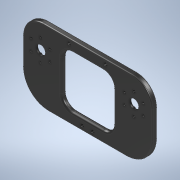
# Autodesk Inventor part: Fechamento_Corpo
Saved by Autodesk Inventor 2020 (Build 240168000, 168)
## iProperties
Created: 2021-05-17
Part Number: Fechamento_Corpo
Material: Plástico PC/ABS
Document SubType Name: Modeling
Designer: JCarlos
Density: 0.357273 g/cm^3
Appearance: Brilhosa - Preta
Author: JCarlos
Autodesk Inventor part; units mm, degrees
ref_plane "YZ Plane" through (0, 0, 0) normal (1, 0, 0) x (0, 1, 0)
ref_plane "XZ Plane" through (0, 0, 0) normal (0, 1, 0) x (-1, 0, 0)
ref_plane "XY Plane" through (0, 0, 0) normal (0, 0, 1) x (1, 0, 0)
sketch "Esboço1" plane through (0, 0, 0) normal (0, 0, 1) x (1, 0, 0)
  line L0 (42.5, 33) -> (-42.5, 33)
  line L1 (-62.5, 13) -> (-62.5, -13)
  line L2 (-37.5, -38) -> (37.5, -38)
  line L3 (62.5, -13) -> (62.5, 13)
  line L4 (-15, 22.5) -> (15, 22.5)
  arc A0 (-15, 22.5) -> (-25, 12.5) centre (-15, 12.5) ccw
  line L5 (-25, -17.5) -> (-25, 12.5)
  arc A1 (-25, -17.5) -> (-15, -27.5) centre (-15, -17.5) ccw
  line L6 (15, -27.5) -> (-15, -27.5)
  arc A2 (15, -27.5) -> (25, -17.5) centre (15, -17.5) ccw
  line L7 (25, 12.5) -> (25, -17.5)
  arc A3 (25, 12.5) -> (15, 22.5) centre (15, 12.5) ccw
  circle A4 centre (-45, 9.5) radius 4.5
  circle A5 centre (-5, -33.75) radius 1.75
  circle A6 centre (5, -33.75) radius 1.75
  circle A7 centre (45, 9.5) radius 4.5
  circle A8 centre (17.5, 28.75) radius 1.75
  circle A9 centre (-17.5, 28.75) radius 1.75
  arc A10 (37.5, -38) -> (62.5, -13) centre (37.5, -13) ccw
  arc A11 (62.5, 13) -> (42.5, 33) centre (42.5, 13) ccw
  arc A12 (-42.5, 33) -> (-62.5, 13) centre (-42.5, 13) ccw
  arc A13 (-62.5, -13) -> (-37.5, -38) centre (-37.5, -13) ccw
  line L8 (0, -38) -> (0, 33)
  line L9 (-76.25, -2.5) -> (83.5363, -2.5)
  point P0 (0, 0)
  point P1 (0, -27.5)
  point P2 (62.5, 0)
  point P3 (0, 22.5)
  point P4 (-62.5, 0)
  dimension "d0" = 125
  dimension "d1" = 71
  dimension "d2" = 25
  dimension "d3" = 20
  dimension "d4" = 9
  dimension "d5" = 3.5
  dimension "d6" = 10
  dimension "d7" = 50
  dimension "d8" = 50
  dimension "d10" = 10.5
  dimension "d11" = 4.25
  dimension "d12" = 10
  dimension "d13" = 5
  dimension "d14" = 35
  dimension "d15" = 17.5
  dimension "d16" = 90
  dimension "d17" = 45
  dimension "d19" = 4.25
  dimension "d77" = 62.5
  dimension "d78" = 71
  dimension "d81" = 10.5
  dimension "d82" = 12
  dimension "d83" = 17.5
  dimension "d84" = 17.5
  constraints: 20 end point, 16 point on circle, 16 tangent, 14 centre point, 9 equal radius, 6 midpoint, 4 horizontal alignment, 2 perpendicular, 2 vertical alignment, 1 horizontal, 1 parallel, 1 point on line
  measures "d0" distance between parallel lines of L1 L3
  measures "d1" distance between parallel lines of L0 L2
  measures "d2" radius of A10
  measures "d3" radius of A11
  measures "d4" diameter of A7
  measures "d5" diameter of A6
  measures "d6" radius of A2
  measures "d7" distance between parallel lines of L5 L7
  measures "d8" distance between parallel lines of L4 L6
  measures "d10" distance between parallel lines of L0 L4
  measures "d11" distance from line of L2 A5.centre
  measures "d12" distance of A5.centre A6.centre
  measures "d13" distance from line of L8 A5.centre
  measures "d14" distance of A9.centre A8.centre
  measures "d15" distance from line of L8 A9.centre
  measures "d16" distance of A4.centre A7.centre
  measures "d17" distance from line of L8 A7.centre
  measures "d19" distance from line of L0 A8.centre
  measures "d77" vertical distance of A5.centre A9.centre
  measures "d78" diameter of L0 L9
  measures "d81" distance between parallel lines of L2 L6
  measures "d82" vertical distance of L9.end A7.centre
  measures "d83" distance from line of L1 A4.centre
  measures "d84" distance from line of L3 A7.centre
extrude "Extrusão1" add sketch "Esboço1" against normal blind 5 contours A11 L3 L9 L7 A3 L4 L8 L0 | L8 L4 A0 L5 L9 L1 A12 L0 | L3 A10 L2 L8 L6 A2 L7 L9 | L9 L5 A1 L6 L8 L2 A13 L1
sketch "Esboço2" plane through (0, 0, -5) normal (0, 0, -1) x (-1, 0, 0)
  circle A0 centre (-45, 9.5) radius 4.5
  line L0 (-48.7227, 17.0463) -> (-47.7691, 23.4146)
  arc A1 (-42.2309, 23.4146) -> (-47.7691, 23.4146) centre (-45, 22.9999) ccw
  arc A2 (-41.2773, 17.0463) -> (-41.2773, 17.0463) centre (-37.585, 11.9538) ccw
  line L1 (-45, 22.9999) -> (-45, -5.684)
  line L2 (-47.6648, 9.5) -> (-30.0023, 9.5)
  circle A3 centre (-45, 9.5) radius 4.5 projected
  circle A4 centre (-45, 9.5) radius 8.4146
  line L3 (-41.2773, 17.0463) -> (-42.2309, 23.4146)
  line L4 (-53.3966, 10.0492) -> (-58.4349, 14.0592)
  arc A5 (-55.6658, 18.8554) -> (-58.4349, 14.0592) centre (-56.6913, 16.25) ccw
  arc A6 (-49.6739, 16.4971) -> (-49.6739, 16.4971) centre (-43.4175, 17.1485) ccw
  line L5 (-49.6739, 16.4971) -> (-55.6658, 18.8554)
  line L6 (-49.6739, 2.5029) -> (-55.6658, 0.1446)
  arc A7 (-58.4349, 4.9408) -> (-55.6658, 0.1446) centre (-56.6913, 2.75) ccw
  arc A8 (-53.3966, 8.9508) -> (-53.3966, 8.9508) centre (-50.8325, 14.6947) ccw
  line L7 (-53.3966, 8.9508) -> (-58.4349, 4.9408)
  line L8 (-41.2773, 1.9537) -> (-42.2309, -4.4146)
  arc A9 (-47.7691, -4.4146) -> (-42.2309, -4.4146) centre (-45, -3.9999) ccw
  arc A10 (-48.7227, 1.9537) -> (-48.7227, 1.9537) centre (-52.415, 7.0462) ccw
  line L9 (-48.7227, 1.9537) -> (-47.7691, -4.4146)
  line L10 (-36.6034, 8.9508) -> (-31.5651, 4.9408)
  arc A11 (-34.3342, 0.1446) -> (-31.5651, 4.9408) centre (-33.3087, 2.75) ccw
  arc A12 (-40.3261, 2.5029) -> (-40.3261, 2.5029) centre (-46.5825, 1.8515) ccw
  line L11 (-40.3261, 2.5029) -> (-34.3342, 0.1446)
  line L12 (-40.3261, 16.4971) -> (-34.3342, 18.8554)
  arc A13 (-31.5651, 14.0592) -> (-34.3342, 18.8554) centre (-33.3087, 16.25) ccw
  arc A14 (-36.6034, 10.0492) -> (-36.6034, 10.0492) centre (-39.1675, 4.3053) ccw
  line L13 (-36.6034, 10.0492) -> (-31.5651, 14.0592)
  arc A15 (-49.6739, 16.4971) -> (-48.7227, 17.0463) centre (-49.4153, 17.1476) ccw
  arc A16 (-53.3966, 8.9508) -> (-53.3966, 10.0492) centre (-53.8307, 9.5) ccw
  arc A17 (-48.7227, 1.9537) -> (-49.6739, 2.5029) centre (-49.4153, 1.8524) ccw
  arc A18 (-40.3261, 2.5029) -> (-41.2773, 1.9537) centre (-40.5847, 1.8524) ccw
  arc A19 (-36.6034, 10.0492) -> (-36.6034, 8.9508) centre (-36.1693, 9.5) ccw
  arc A20 (-41.2773, 17.0463) -> (-40.3261, 16.4971) centre (-40.5847, 17.1476) ccw
  point P0 (0, 0)
  point P1 (19.7723, -33.3719)
  point P2 (-53.3966, 8.9508)
  point P3 (-49.6739, 2.5029)
  point P4 (-48.7227, 1.9537)
  point P5 (-41.2773, 1.9537)
  point P6 (-40.3261, 2.5029)
  point P7 (-36.6034, 8.9508)
  point P8 (-36.6034, 10.0492)
  point P9 (-40.3261, 16.4971)
  point P10 (-41.2773, 17.0463)
  point P11 (-49.6739, 16.4971)
  point P12 (-53.3966, 10.0492)
  dimension "d22" = 2.8
  dimension "d24" = 13.4999
  dimension "d31" = 8.516
  dimension "d35" = 16.8291
  dimension "d36" = 8.516
  dimension "d37" = 3.7227
  dimension "d40" = 360
  dimension "d42" = 0.7
  dimension "d45" = 360
  dimension "d47" = 3.7227
  dimension "d48" = 5.8515
  constraints: 40 end point, 39 point on circle, 20 centre point, 2 concentric, 2 point on line, 1 coincident, 1 horizontal, 1 horizontal alignment, 1 perpendicular, 1 tangent, 1 vertical, 92 other
  measures "d22" radius of A1
  measures "d24" distance of A0.centre L1.start
  measures "d31" angle of L1 L0
  measures "d35" diameter of A4
  measures "d36" angle of L3 L1
  measures "d37" horizontal distance of L1.start L0.start
  measures "d42" radius of A15
  measures "d47" horizontal distance of L3.start L1.start
  measures "d48" vertical distance of L1.start A6.centre
extrude "Extrusão2" cut sketch "Esboço2" against normal blind 2.5 contours L2 A19 A4 A2 A0 | A0 A14 A19 L2 | A0 A6 A4 A14 | A2 A4 A12 A0 | A0 A2 A20 A4 A6 | A4 A6 L12 A2 L13 | A12 A18 A4 A14 L1 A0 | A4 L10 A2 | A2 L10 A14 L11 A4 | A0 A8 L1 A4 A2 | A4 L12 A6 | A2 L12 A13 L13 | L1 A14 A0 | A0 L1 A8 | A4 A8 L0 A6 L3 | A14 L1 A4 A10 A0 | A14 A4 L1 | L8 A14 A4 | A14 L10 A11 L11 | A0 A6 A15 A4 A8 L1 | L1 A8 A4 | A6 L0 A1 L3 | A10 A17 A4 A12 A0 | A4 A14 L8 A12 L1 | L1 A12 L9 A4 | A0 A10 A4 A6 | A4 L0 A8 | A12 A4 A8 A0 | A12 L8 A9 L9 | A8 A16 A4 A10 A0 | A4 A10 L4 A8 L5 | A12 L6 A10 L7 A4 | A4 L6 A12 | A4 L4 A10 | A8 L4 A5 L5 | L6 A7 L7 A10 picked at (-45.103, 3.2982) picked at (-44.9157, 15.7791)
sketch "Esboço3" plane through (0, 0, -5) normal (0, 0, -1) x (-1, 0, 0)
  circle A0 centre (-17.5, 28.75) radius 1.75 projected
  point P0 (0, 0)
  constraints: 1 coincident
hole "Furo1" at (17.5, 28.75, -5) direction (0, 0, 1) diameter 6 depth 2.5
sketch "Esboço4" plane through (0, 0, -5) normal (0, 0, -1) x (-1, 0, 0)
  circle A0 centre (-5, -33.75) radius 1.75 projected
  point P0 (0, 0)
  constraints: 1 coincident
hole "Furo2" at (5, -33.75, -5) direction (0, 0, 1) diameter 6 depth 2.5
mirror "Espelhamento1" about plane through (0, 0, 0) normal (1, 0, 0) of "Extrusão2", "Furo1", "Furo2"
fillet "Arredondamento1" radius 2 16 edges at (0, 22.5, 0) (22.0711, 19.5711, 0) (25, -2.5, 0) (22.0711, -24.5711, 0) (0, -27.5, 0) (-22.0711, -24.5711, 0) (-25, -2.5, 0) (-22.0711, 19.5711, 0) (-22.0711, -24.5711, -5) (0, -27.5, -5) (22.0711, -24.5711, -5) (25, -2.5, -5) (22.0711, 19.5711, -5) (0, 22.5, -5) (-22.0711, 19.5711, -5) (-25, -2.5, -5)
fillet "Arredondamento1" radius 1 16 edges at (-56.6421, 27.1421, 0) (-62.5, 0, 0) (-55.1777, -30.6777, 0) (0, -38, 0) (55.1777, -30.6777, 0) (62.5, 0, 0) (56.6421, 27.1421, 0) (0, 33, 0) (56.6421, 27.1421, -5) (62.5, 0, -5) (55.1777, -30.6777, -5) (0, -38, -5) (-55.1777, -30.6777, -5) (-62.5, 0, -5) (-56.6421, 27.1421, -5) (0, 33, -5)
chamfer "Chanfro1" distance 1 angle 45 2 edges at (40.5, 9.5, -2.5) (-49.5, 9.5, -2.5)
sketch "Esboço5" plane through (0, 0, -2.5) normal (0, 0, -1) x (-1, 0, 0)
  circle A0 centre (-45, 9.5) radius 10.5
  circle A1 centre (-45, 9.5) radius 4.5 projected
  circle A2 centre (-35.9067, 14.75) radius 1.25
  line L0 (-45, 9.5) -> (-33.3087, 16.25)
  arc A3 (-31.5651, 14.0592) -> (-34.3342, 18.8554) centre (-33.3087, 16.25) ccw projected
  point P0 (0, 0)
  dimension "d70" = 21
  dimension "d71" = 2.5
  constraints: 2 end point, 1 centre point, 1 coincident, 1 point on line, 4 other
  measures "d71" diameter of A2
extrude "Extrusão3" cut sketch "Esboço5" against normal through all contours A2 L0 A0 | A0 L0 A2 | A2 L0 A0 | A0 L0 A2
pattern_circular "Padrão circular1" count 6 over 360 about axis through (45, 9.5, 0) along (0, 0, -1) of "Extrusão3"
mirror "Espelhamento2" about plane through (0, 0, 0) normal (1, 0, 0) of "Extrusão3", "Padrão circular1"
equation "\"d11\" = d19"
equation "\"d15\" = 0.5 * d14"
equation "\"d17\" = 0.5 * d16"
equation "\"d78\" = d1"
equation "\"d81\" = -0.5 * d8 + 0.5 * d1"
